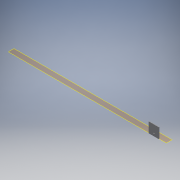
# Autodesk Inventor part: block
Saved by Autodesk Inventor 2016 (Build 200138000, 138)
## iProperties
Created: 2016-03-19
Part Number: block
Material: Generic
Document SubType Name: Modeling
Designer: gus
Density: 1 g/cm^3
Appearance: Default
Author: gus
Autodesk Inventor part; units mm, degrees
ref_plane "YZ Plane" through (0, 0, 0) normal (1, 0, 0) x (0, 1, 0)
ref_plane "XZ Plane" through (0, 0, 0) normal (0, 1, 0) x (-1, 0, 0)
ref_plane "XY Plane" through (0, 0, 0) normal (0, 0, 1) x (1, 0, 0)
ref_plane "Work Plane1" through (0, 50.8, 0) normal (0, 1, 0) x (0, 0, -1)
sketch "Sketch1" plane through (0, 50.8, 0) normal (0, 1, 0) x (0, 0, -1)
  line L0 (0, 50.8) -> (-25.4, 50.8)
  line L1 (-25.4, 50.8) -> (-25.4, 0)
  line L2 (-25.4, 0) -> (0, 0)
  line L3 (0, 0) -> (0, 50.8)
  line L4 (-3.175, 3.175) -> (-22.225, 3.175)
  line L5 (-22.225, 3.175) -> (-22.225, 47.625)
  line L6 (-22.225, 47.625) -> (-3.175, 47.625)
  line L7 (-3.175, 47.625) -> (-3.175, 3.175)
  point P0 (0, 0)
  dimension "d0" = 25.4
  dimension "d1" = 50.8
  dimension "d9" = 3.175
  constraints: 16 end point, 4 parallel, 2 perpendicular, 1 coincident, 1 horizontal, 3 other
  measures "d0" distance of L2.end L1.end
  measures "d1" distance of L1.end L0.end
  measures "d9" distance between parallel lines of L2 L4
extrude "Extrusion3" add sketch "Sketch1" along normal blind 50.8
sketch "Sketch3" plane through (-50.8, 50.8, 25.4) normal (0, 0, 1) x (1, 0, 0)
  circle A0 centre (25.4, 12.7) radius 3.3734
  line L0 (0, 0) -> (50.8, 0) projected
  line L1 (0, 0) -> (0, 50.8) projected
  line L2 (41.275, 38.1) -> (41.275, 12.7) construction
  line L3 (38.1, 38.1) -> (38.1, 12.7)
  line L4 (44.45, 12.7) -> (44.45, 38.1)
  arc A1 (44.45, 38.1) -> (38.1, 38.1) centre (41.275, 38.1) ccw
  arc A2 (38.1, 12.7) -> (44.45, 12.7) centre (41.275, 12.7) ccw
  line L5 (50.8, 0) -> (50.8, 50.8) projected
  line L6 (3.175, 0) -> (47.625, 0) construction
  line L7 (25.4, 0) -> (25.4, 50.8) construction
  line L8 (47.625, 50.8) -> (3.175, 50.8) construction
  line L9 (12.7, 38.1) -> (12.7, 12.7)
  line L10 (6.35, 12.7) -> (6.35, 38.1)
  arc A3 (12.7, 38.1) -> (6.35, 38.1) centre (9.525, 38.1) ccw
  arc A4 (6.35, 12.7) -> (12.7, 12.7) centre (9.525, 12.7) ccw
  point P0 (50.8, -50.8)
  point P1 (41.275, 25.4)
  dimension "d12" = 6.7469
  dimension "d13" = 12.7
  dimension "d14" = 25.4
  dimension "d20" = 6.35
  dimension "d21" = 25.4
  dimension "d22" = 9.525
  dimension "d23" = 25.4
  constraints: 14 end point, 8 point on circle, 6 symmetric about line, 5 centre point, 4 tangent, 3 midpoint, 1 parallel, 1 vertical, 2 other
  measures "d12" diameter of A0
  measures "d13" distance from line of L0 A0.centre
  measures "d14" distance from line of L1 A0.centre
  measures "d20" diameter of A2
  measures "d21" distance of L2.end L2.start
  measures "d22" distance from line of L5 point (41.275, 25.4)
  measures "d23" distance from line of L0 point (41.275, 25.4)
extrude "Extrusion4" cut sketch "Sketch3" against normal blind 25.4
sketch "Sketch4" plane through (0, 50.8, 25.4) normal (1, 0, 0) x (0, 0, -1)
  line L0 (3.175, 0) -> (3.175, 50.8) projected
  line L1 (22.225, 0) -> (22.225, 50.8) projected
  line L2 (3.175, 0) -> (22.225, 0)
  line L3 (22.225, 0) -> (22.225, 25.4)
  line L4 (22.225, 25.4) -> (3.175, 25.4)
  line L5 (3.175, 25.4) -> (3.175, 0)
  point P0 (25.4, -50.8)
  dimension "d17" = 25.4
  constraints: 8 end point, 2 parallel, 1 horizontal, 1 midpoint, 1 perpendicular
  measures "d17" distance between parallel lines of L2 L4
extrude "Extrusion5" cut sketch "Sketch4" against normal blind 50.8
body "Solid2"
